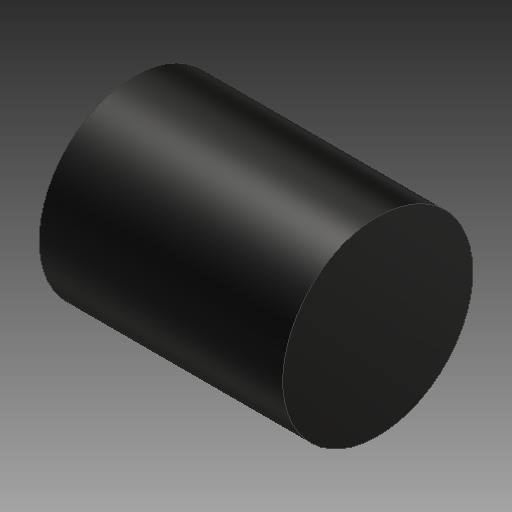
# Autodesk Inventor part: Encoder
Saved by Autodesk Inventor 2018 (Build 220112000, 112)
## iProperties
Created: 2018-09-18
Part Number: Encoder
Material: Generic
Document SubType Name: Modeling
Designer: Viraj Shah
Density: 1 g/cm^3
Appearance: Default
Mass: 4.12177 g
Surface Area: 14.3257 cm^2
Volume: 4.12177 cm^3
Author: Viraj Shah
Autodesk Inventor part; units mm, degrees
ref_plane "YZ Plane" through (0, 0, 0) normal (1, 0, 0) x (0, 1, 0)
ref_plane "XZ Plane" through (0, 0, 0) normal (0, 1, 0) x (-1, 0, 0)
ref_plane "XY Plane" through (0, 0, 0) normal (0, 0, 1) x (1, 0, 0)
sketch "Sketch1" plane through (0, 0, 0) normal (1, 0, 0) x (0, 1, 0)
  circle A0 centre (0, -0.2568) radius 8
  point P0 (0, 0)
  dimension "d0" = 16
  constraints: 1 centre point
  measures "d0" diameter of A0
extrude "Extrusion1" add sketch "Sketch1" along normal blind 20.5
body "Solid1"
